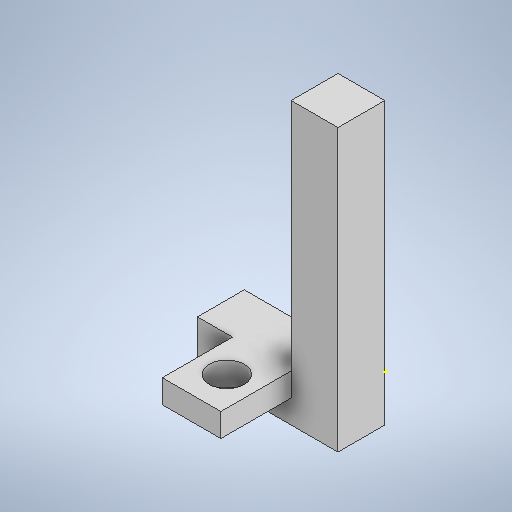
# Autodesk Inventor part: steering_helper_base[1]
Saved by Autodesk Inventor 2025.2 (Build 292293000, 293)
## iProperties
Created: 2025-02-06
Part Number: steering_helper_base[1]
Material: Generic
Document SubType Name: Modeling
Designer: mpava
Density: 1 g/cm^3
Appearance: Default
Author: mpava
Autodesk Inventor part; units mm, degrees
ref_plane "YZ Plane" through (0, 0, 0) normal (1, 0, 0) x (0, 1, 0)
ref_plane "XZ Plane" through (0, 0, 0) normal (0, 1, 0) x (-1, 0, 0)
ref_plane "XY Plane" through (0, 0, 0) normal (0, 0, 1) x (1, 0, 0)
sketch "Sketch1" plane through (0, 0, 0) normal (0, 0, 1) x (1, 0, 0)
  line L0 (0, 60) -> (0, -60)
  line L1 (0, 60) -> (-20, 60)
  line L2 (-20, 60) -> (-20, -40)
  line L3 (-20, -40) -> (-60, -40)
  line L4 (-60, -40) -> (-60, -60)
  line L5 (-60, -60) -> (0, -60)
  point P0 (0, 0)
  dimension "d0" = 120
  dimension "d1" = 20
  dimension "d2" = 100
  dimension "d3" = 40
  dimension "d4" = 20
  constraints: 12 end point, 2 perpendicular, 1 horizontal, 1 midpoint, 1 parallel, 1 vertical
  measures "d0" distance of L0.start L0.end
  measures "d1" distance of L0.start L1.end
  measures "d2" distance of L1.end L2.end
  measures "d3" distance of L2.end L3.end
  measures "d4" distance of L3.end L4.end
extrude "Extrusion1" add sketch "Sketch1" along normal blind 20
sketch "Sketch2" plane through (0, 0, 20) normal (0, 0, 1) x (1, 0, 0)
  line L0 (-20, -40) -> (-60, -40) projected
  line L1 (-20, -40) -> (-20, -50)
  line L2 (-20, -50) -> (-45, -50)
  line L3 (-45, -50) -> (-45, -40)
  point P0 (0, 0)
  dimension "d7" = 10
  dimension "d8" = 25
  constraints: 6 end point, 2 perpendicular, 1 point on line, 1 vertical
  measures "d7" distance of L0.start L1.end
  measures "d8" distance of L1.end L2.end
extrude "Extrusion2" add sketch "Sketch2" along normal blind 30
sketch "Sketch3" plane through (-60, -40, 0) normal (0, 1, 0) x (1, 0, 0)
  point P0 (60, 0)
sketch "Sketch4" plane through (-60, -40, 0) normal (0, 1, 0) x (1, 0, 0)
  line L0 (40, -50) -> (15, -50) projected
  line L1 (40, -20) -> (40, -50) projected
  circle A0 centre (27.5, -35) radius 7.5
  point P0 (60, 0)
  dimension "d11" = 15
  constraints: 1 centre point
  measures "d11" diameter of A0
extrude "Extrusion3" cut sketch "Sketch4" against normal blind 10
body "Solid1"
